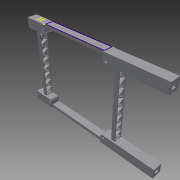
# Autodesk Inventor part: NUCholder
Saved by Autodesk Inventor 2015 (Build 190159000, 159)
## iProperties
Created: 2015-04-17
Part Number: NUCholder
Material: Generic
Document SubType Name: Modeling
Designer: Akovo_000
Density: 1 g/cm^3
Appearance: Default
Author: Akovo_000
Autodesk Inventor part; units mm, degrees
ref_plane "YZ Plane" through (0, 0, 0) normal (1, 0, 0) x (0, 1, 0)
ref_plane "XZ Plane" through (0, 0, 0) normal (0, 1, 0) x (-1, 0, 0)
ref_plane "XY Plane" through (0, 0, 0) normal (0, 0, 1) x (1, 0, 0)
sketch "Button Layer" plane through (0, 0, 0) normal (0, 1, 0) x (-1, 0, 0)
  line L0 (-73.3766, -28.1226) -> (16.7234, -28.1226)
  circle A0 centre (16.7234, -28.1226) radius 1.5
  circle A1 centre (-73.3766, -28.1226) radius 1.5
  line L1 (16.7234, 2.8734) -> (-73.3766, 2.8734)
  circle A2 centre (-11.2766, 30.8734) radius 28
  line L2 (-73.3766, 2.8734) -> (-73.3766, -28.1226)
  line L3 (-73.3766, 47.3774) -> (-73.3766, 2.8734)
  line L4 (16.7234, 2.8734) -> (16.7234, 58.8734)
  line L5 (16.7234, 2.8734) -> (16.7234, -28.1226)
  circle A3 centre (9.7234, -21.1226) radius 3
  circle A4 centre (9.7234, -21.1226) radius 2.5
  line L6 (9.7234, -21.1226) -> (16.7234, -21.1226)
  line L7 (16.7234, -21.1226) -> (16.7234, -28.1226)
  line L8 (16.7234, -28.1226) -> (9.7234, -28.1226)
  line L9 (9.7234, -28.1226) -> (9.7234, -21.1226)
  line L10 (9.7234, -21.1226) -> (-2.2766, -21.1226)
  line L11 (-2.2766, -21.1226) -> (-2.2766, -15.6226)
  line L12 (-2.2766, -15.6226) -> (9.7234, -15.6226)
  line L13 (9.7234, -15.6226) -> (9.7234, -21.1226)
  circle A5 centre (9.7234, -15.6226) radius 2.5
  circle A6 centre (-2.2766, -15.6226) radius 2.5
  line L14 (15.1646, -25.4226) -> (18.2823, -25.4226)
  line L15 (18.2823, -25.4226) -> (19.8411, -28.1226)
  line L16 (19.8411, -28.1226) -> (18.2823, -30.8226)
  line L17 (18.2823, -30.8226) -> (15.1646, -30.8226)
  line L18 (15.1646, -30.8226) -> (13.6057, -28.1226)
  line L19 (13.6057, -28.1226) -> (15.1646, -25.4226)
  line L20 (-74.9354, -25.4226) -> (-71.8177, -25.4226)
  line L21 (-71.8177, -25.4226) -> (-70.2589, -28.1226)
  line L22 (-70.2589, -28.1226) -> (-71.8177, -30.8226)
  line L23 (-71.8177, -30.8226) -> (-74.9354, -30.8226)
  line L24 (-74.9354, -30.8226) -> (-76.4943, -28.1226)
  line L25 (-76.4943, -28.1226) -> (-74.9354, -25.4226)
  line L26 (16.7234, 79.3734) -> (-73.3766, 79.3734)
  line L27 (-73.3766, -15.6266) -> (16.7234, -15.6266)
  circle A7 centre (16.7234, 79.3734) radius 1.5
  circle A8 centre (16.7234, -15.6266) radius 1.5
  circle A9 centre (-73.3766, -15.6266) radius 1.5
  circle A10 centre (-73.3766, 79.3734) radius 1.5
  line L28 (-73.3766, 59.8734) -> (16.7234, 59.8734)
  line L29 (-73.3766, 3.8734) -> (-73.3766, -15.6266)
  line L30 (-73.3766, 59.8734) -> (-73.3766, 79.3734)
  line L31 (-73.3766, 59.8734) -> (-73.3766, 3.8734)
  line L32 (16.7234, 3.8734) -> (16.7234, 59.8734)
  line L33 (16.7234, 3.8734) -> (16.7234, -15.6266)
  circle A11 centre (9.7234, -8.6266) radius 3
  circle A12 centre (9.7234, -8.6266) radius 2.5
  line L34 (9.7234, -8.6266) -> (16.7234, -8.6266)
  line L35 (16.7234, -8.6266) -> (16.7234, -15.6266)
  line L36 (16.7234, -15.6266) -> (9.7234, -15.6266)
  line L37 (9.7234, -15.6266) -> (9.7234, -8.6266)
  line L38 (9.7234, -8.6266) -> (-2.2766, -8.6266)
  line L39 (-2.2766, -8.6266) -> (-2.2766, -3.1266)
  line L40 (-2.2766, -3.1266) -> (9.7234, -3.1266)
  line L41 (9.7234, -3.1266) -> (9.7234, -8.6266)
  circle A13 centre (9.7234, -3.1266) radius 2.5
  circle A14 centre (-2.2766, -3.1266) radius 2.5
  line L42 (15.1646, -12.9266) -> (18.2823, -12.9266)
  line L43 (18.2823, -12.9266) -> (19.8411, -15.6266)
  line L44 (19.8411, -15.6266) -> (18.2823, -18.3266)
  line L45 (18.2823, -18.3266) -> (15.1646, -18.3266)
  line L46 (15.1646, -18.3266) -> (13.6057, -15.6266)
  line L47 (13.6057, -15.6266) -> (15.1646, -12.9266)
  line L48 (15.1646, 82.0734) -> (18.2823, 82.0734)
  line L49 (18.2823, 82.0734) -> (19.8411, 79.3734)
  line L50 (19.8411, 79.3734) -> (18.2823, 76.6734)
  line L51 (18.2823, 76.6734) -> (15.1646, 76.6734)
  line L52 (15.1646, 76.6734) -> (13.6057, 79.3734)
  line L53 (13.6057, 79.3734) -> (15.1646, 82.0734)
  line L54 (-74.9354, 82.0734) -> (-71.8177, 82.0734)
  line L55 (-71.8177, 82.0734) -> (-70.2589, 79.3734)
  line L56 (-70.2589, 79.3734) -> (-71.8177, 76.6734)
  line L57 (-71.8177, 76.6734) -> (-74.9354, 76.6734)
  line L58 (-74.9354, 76.6734) -> (-76.4943, 79.3734)
  line L59 (-76.4943, 79.3734) -> (-74.9354, 82.0734)
  line L60 (-74.9354, -12.9266) -> (-71.8177, -12.9266)
  line L61 (-71.8177, -12.9266) -> (-70.2589, -15.6266)
  line L62 (-70.2589, -15.6266) -> (-71.8177, -18.3266)
  line L63 (-71.8177, -18.3266) -> (-74.9354, -18.3266)
  line L64 (-74.9354, -18.3266) -> (-76.4943, -15.6266)
  line L65 (-76.4943, -15.6266) -> (-74.9354, -12.9266)
  line L66 (41.6234, -38.1226) -> (-138.3766, -38.1226)
  line L67 (-138.3766, -38.1226) -> (-138.3766, 63.8774)
  line L68 (-138.3766, 63.8774) -> (41.6234, 63.8774)
  line L69 (41.6234, 63.8774) -> (41.6234, -38.1226)
  circle A15 centre (-73.3766, -15.6266) radius 3.5
  circle A16 centre (16.7234, -15.6266) radius 3.5
  circle A17 centre (-73.3766, 79.3734) radius 3.5
  circle A18 centre (16.7234, 79.3734) radius 3.5
  line L70 (41.6234, -38.1226) -> (13.2234, -38.1226)
  line L71 (13.2234, -38.1226) -> (13.2234, -12.1266)
  line L72 (13.2234, -12.1266) -> (41.6234, -12.1266)
  line L73 (41.6234, -12.1266) -> (41.6234, -38.1226)
  line L74 (-138.3766, -38.1226) -> (-69.8766, -38.1226)
  line L75 (-69.8766, -38.1226) -> (-69.8766, -12.1266)
  line L76 (-69.8766, -12.1266) -> (-138.3766, -12.1266)
  line L77 (-138.3766, -12.1266) -> (-138.3766, -38.1226)
  line L78 (16.7234, 59.8734) -> (16.7234, 79.3734)
  point P0 (0, 0)
  point P1 (0, 0)
  point P2 (0, 0)
  dimension "d33" = 90.1
  dimension "d35" = 6
  dimension "d36" = 0.5
  dimension "d37" = 5
  dimension "d38" = 12
  dimension "d39" = 7
  dimension "d40" = 5.4
  dimension "d41" = 3
  dimension "d43" = 90.1
  dimension "d45" = 6
  dimension "d46" = 0.5
  dimension "d47" = 5
  dimension "d48" = 12
  dimension "d49" = 7
  dimension "d50" = 5.4
  dimension "d63" = 180
  dimension "d64" = 102
  dimension "d65" = 65
  dimension "d66" = 24.9
  dimension "d67" = 22.496
  dimension "d68" = 7
  dimension "d69" = 10
  dimension "d70" = 57
  constraints: 158 end point, 20 coincident, 19 centre point, 15 parallel, 10 perpendicular, 9 equal length, 9 horizontal, 8 equal radius, 8 tangent, 5 collinear, 4 vertical, 2 concentric, 78 other
  measures "d33" distance of L0.start L0.end
  measures "d35" diameter of A3
  measures "d36" radial gap between concentric circles of A3 A4
  measures "d37" diameter of A5
  measures "d38" distance between parallel lines of L11 L13
  measures "d39" distance of L6.start L6.end
  measures "d40" distance between parallel lines of L15 L18
  measures "d41" diameter of A7
  measures "d43" distance of L27.start L27.end
  measures "d45" diameter of A11
  measures "d46" radial gap between concentric circles of A11 A12
  measures "d47" diameter of A13
  measures "d48" distance between parallel lines of L39 L41
  measures "d49" distance of L34.start L34.end
  measures "d50" distance between parallel lines of L43 L46
  measures "d63" distance of L67.end L68.end
  measures "d64" distance of L66.end L67.end
  measures "d65" distance between parallel lines of L67 L29
  measures "d66" distance between parallel lines of L69 L32
  measures "d67" distance between parallel lines of L66 L27
  measures "d68" diameter of A15
  measures "d69" distance between parallel lines of L66 L0
  measures "d70" distance between parallel lines of L28 L1
sketch "NucSupport" plane through (0, 0, 0) normal (0, 1, 0) x (-1, 0, 0)
  line L0 (0, 0) -> (-180, 0)
  line L1 (-180, 0) -> (-180, 110)
  line L2 (-180, 110) -> (0, 110)
  line L3 (0, 110) -> (0, 0)
  line L4 (-24.9, 8.5) -> (-115, 8.5)
  line L5 (-115, 8.5) -> (-115, 101.5)
  line L6 (-115, 101.5) -> (-24.9, 101.5)
  line L7 (-24.9, 101.5) -> (-24.9, 8.5)
  line L8 (-24.9, 12) -> (0, 12)
  line L9 (-28.4, 8.5) -> (-28.4, 0)
  line L10 (-24.9, 98) -> (0, 98)
  line L11 (-28.4, 101.5) -> (-28.4025, 110)
  line L12 (-111.5, 101.5) -> (-111.5, 110)
  line L13 (-115, 98) -> (-180, 98)
  line L14 (-115, 12) -> (-180, 12)
  line L15 (-111.5, 8.5) -> (-111.5, 0)
  circle A0 centre (-115, 8.5) radius 3.5
  circle A1 centre (-24.9, 8.5) radius 3.5
  circle A2 centre (-115, 101.5) radius 3.5
  circle A3 centre (-24.9, 101.5) radius 3.5
  dimension "d174" = 7
  dimension "d71" = 180
  dimension "d72" = 110
  dimension "d73" = 90.1
  dimension "d74" = 93
  dimension "d75" = 65
  dimension "d176" = 24.9
  constraints: 32 end point, 16 point on line, 9 equal length, 4 coincident, 4 horizontal, 3 vertical, 2 horizontal alignment, 2 vertical alignment, 1 perpendicular, 9 other
  measures "d71" distance of L0.start L0.end
  measures "d72" distance of L0.end L1.end
  measures "d73" distance of L5.end L6.end
  measures "d74" distance of L4.end L5.end
  measures "d75" distance between parallel lines of L1 L5
  measures "d176" distance between parallel lines of L3 L7
extrude "NucSupportHorizontal" add sketch "NucSupport" along normal blind 2 contours L0 L9 A1 L8 L3 | L0 L1 L14 A0 L15 | A1 L7 L4 | L4 L7 A1 | L10 A3 L11 L2 L3 | A0 L5 L4 | L4 L5 A0 | A3 L6 L7 | L7 L6 A3 | L1 L2 L12 A2 L13 | A2 L6 L5 | L5 L6 A2
sketch "Sketch4" plane through (0, 2, 0) normal (0, 1, 0) x (1, 0, 0)
  arc A0 (28.4, -101.5) -> (24.9, -98) centre (24.9, -101.5) ccw projected
  circle A1 centre (24.9, -101.5) radius 3.5
  arc A2 (115, -98) -> (111.5, -101.5) centre (115, -101.5) ccw projected
  circle A3 centre (115, -101.5) radius 3.5
  arc A4 (111.5, -8.5) -> (115, -12) centre (115, -8.5) ccw projected
  circle A5 centre (115, -8.5) radius 3.5
  arc A6 (24.9, -12) -> (28.4, -8.5) centre (24.9, -8.5) ccw projected
  circle A7 centre (24.9, -8.5) radius 3.5
  constraints: 7 equal radius, 4 centre point, 4 coincident
hole "Holes" at (24.9, 2, 101.5) at (24.9, 2, 8.5) at (115, 2, 8.5) at (115, 2, 101.5) direction (0, -1, 0) diameter 3.5 depth 7
sketch "Sketch6" plane through (0, 2, 0) normal (0, 1, 0) x (1, 0, 0)
  line L0 (0, 0) -> (28.4, 0)
  line L1 (28.4, 0) -> (28.4, -8.5)
  line L2 (28.4, -8.5) -> (28.4, 0) projected
  line L3 (24.9, -12) -> (0, -12)
  line L4 (0, -12) -> (0, 0)
  line L5 (0, 0) -> (0, -12) projected
  line L6 (0, -98) -> (24.9, -98)
  line L7 (24.9, -98) -> (0, -98) projected
  line L8 (0, -110) -> (28.4025, -110) projected
  line L9 (28.4025, -110) -> (0, -110)
  line L10 (0, -110) -> (0, -98)
  line L11 (111.5, -110) -> (111.5, -101.5)
  arc A0 (115, -98) -> (111.5, -101.5) centre (115, -101.5) ccw projected
  line L12 (115, -98) -> (180, -98)
  line L13 (180, -98) -> (115, -98) projected
  line L14 (180, -98) -> (180, -110)
  line L15 (180, -110) -> (111.5, -110)
  line L16 (111.5, 0) -> (180, 0)
  line L17 (180, 0) -> (111.5, 0) projected
  line L18 (180, 0) -> (180, -12)
  line L19 (180, -12) -> (115, -12)
  arc A1 (111.5, -8.5) -> (115, -12) centre (115, -8.5) ccw projected
  line L20 (111.5, -8.5) -> (111.5, 0)
  circle A2 centre (115, -101.5) radius 1.75 projected
  arc A3 (115, -98) -> (111.5, -101.5) centre (115, -101.5) ccw
  circle A4 centre (24.9, -8.5) radius 1.75 projected
  arc A5 (24.9, -12) -> (28.4, -8.5) centre (24.9, -8.5) ccw
  circle A6 centre (115, -8.5) radius 1.75 projected
  arc A7 (111.5, -8.5) -> (115, -12) centre (115, -8.5) ccw
  circle A8 centre (24.9, -101.5) radius 1.75 projected
  arc A9 (28.4, -101.5) -> (24.9, -98) centre (24.9, -101.5) ccw
  arc A10 (28.4, -101.5) -> (24.9, -98) centre (24.9, -101.5) ccw projected
  line L21 (28.4, -101.5) -> (28.4025, -110)
  line L22 (0, -12) -> (24.9, -12) projected
  line L23 (28.4025, -110) -> (28.4, -101.5) projected
  line L24 (111.5, -101.5) -> (111.5, -110) projected
  line L25 (111.5, 0) -> (111.5, -8.5) projected
  line L26 (16.9, -12) -> (16.9, -98)
  line L27 (11.9, -98) -> (11.9, -12)
  line L28 (125, -12) -> (125, -98)
  line L29 (180, -98) -> (115, -98) projected
  line L30 (115, -12) -> (180, -12) projected
  line L31 (130, -12) -> (130, -98)
  line L32 (28.4, 0) -> (111.5, 0)
  line L33 (111.5, 0) -> (111.5, -4.25)
  line L34 (111.5, -4.25) -> (28.4, -4.25)
  line L35 (28.4, -4.25) -> (28.4, 0)
  line L36 (111.5, -110) -> (28.4013, -110)
  line L37 (28.4013, -110) -> (28.4013, -105.75)
  line L38 (28.4013, -105.75) -> (111.5, -105.75)
  line L39 (111.5, -105.75) -> (111.5, -110)
  dimension "d179" = 5
  dimension "d181" = 5
  dimension "d183" = 8
  dimension "d184" = 10
  constraints: 56 end point, 9 perpendicular, 9 point on line, 8 point on circle, 7 parallel, 6 collinear, 5 tangent, 4 centre point, 4 coincident, 3 horizontal, 2 midpoint, 1 vertical
  measures "d179" distance between parallel lines of L27 L26
  measures "d181" distance between parallel lines of L31 L28
  measures "d183" distance from line of L26 A5.centre
  measures "d184" distance from line of A7.centre L28
extrude "Big Holder" add sketch "Sketch6" along normal blind 10 contours L0 L1 A5 L3 L4 | L32 L20 L34 L1 | L16 L18 L19 A1 L20 | L3 L26 L6 L27 | L6 A9 L21 L8 L10 | L31 L12 L28 L19 | L12 L14 L15 L11 A0 | L21 L38 L11 L36
sketch "Air Grill" plane through (130, 2, 98) normal (1, 0, 0) x (0, 0, -1)
  line L0 (0, 10) -> (86, 10)
  line L1 (86, 10) -> (86, 0)
  line L2 (86, 0) -> (0, 0)
  line L3 (0, 0) -> (0, 10)
  line L4 (1, 10) -> (85, 10)
  line L5 (85, 10) -> (85, 9.1738)
  line L6 (1, 9.1738) -> (1, 10)
  line L7 (0, 0) -> (86, 0) projected
  line L8 (1, 0) -> (85, 0)
  line L9 (85, 0) -> (85, 1.1182)
  line L10 (1, 0.8262) -> (1, 0)
  line L11 (89.5, 10) -> (86, 10) projected
  line L12 (1, 9.1738) -> (1, 0.8262)
  line L13 (85, 9.1738) -> (85, 1.1182)
  line L14 (86, 0) -> (86, 10) projected
  line L15 (1, 9.1738) -> (5.6509, 1.1182)
  line L16 (1, 9.1738) -> (10.3019, 9.1738) construction
  line L17 (6.4592, 1.1182) -> (11.1102, 9.1738)
  line L18 (6.4592, 1.1182) -> (15.7611, 1.1182) construction
  line L19 (11.9184, 9.1738) -> (16.5694, 1.1182)
  line L20 (17.3777, 1.1182) -> (22.0286, 9.1738)
  line L21 (17.3777, 1.1182) -> (26.6795, 1.1182) construction
  line L22 (22.8369, 9.1738) -> (28.3475, 1.1182)
  line L23 (29.1558, 1.1182) -> (33.8068, 9.1738)
  line L24 (29.1558, 1.1182) -> (38.4577, 1.1182) construction
  line L25 (34.6151, 9.1738) -> (39.266, 1.1182)
  line L26 (34.6151, 9.1738) -> (43.9169, 9.1738) construction
  line L27 (40.0743, 1.1182) -> (44.1917, 9.1738)
  line L28 (11.9184, 9.1738) -> (7.801, 1.1182)
  line L29 (12.7267, 9.1738) -> (17.3777, 1.1182)
  line L30 (18.7195, 1.1182) -> (22.8369, 9.1738)
  line L31 (24.5049, 9.1738) -> (29.1558, 1.1182)
  line L32 (30.4976, 1.1182) -> (34.6151, 9.1738)
  line L33 (35.4234, 9.1738) -> (40.0743, 1.1182)
  line L34 (40.8826, 1.1182) -> (45, 9.1738)
  line L35 (6.4592, 1.1182) -> (5.6509, 1.1182)
  line L36 (16.5694, 1.1182) -> (17.3777, 1.1182)
  line L37 (11.1102, 9.1738) -> (11.9184, 9.1738)
  line L38 (11.9184, 9.1738) -> (11.9184, 9.1738)
  line L39 (12.7267, 9.1738) -> (11.9184, 9.1738)
  line L40 (12.7267, 9.1738) -> (22.0286, 9.1738)
  line L41 (22.0286, 9.1738) -> (22.8369, 9.1738)
  line L42 (22.8369, 9.1738) -> (22.8369, 9.1738)
  line L43 (22.8369, 9.1738) -> (24.5049, 9.1738)
  line L44 (33.8068, 9.1738) -> (24.5049, 9.1738)
  line L45 (33.8068, 9.1738) -> (34.6151, 9.1738)
  line L46 (34.6151, 9.1738) -> (34.6151, 9.1738)
  line L47 (35.4234, 9.1738) -> (34.6151, 9.1738)
  line L48 (35.4234, 9.1738) -> (44.1917, 9.1738)
  line L49 (45, 9.1738) -> (44.1917, 9.1738)
  line L50 (17.3777, 1.1182) -> (17.3777, 1.1182)
  line L51 (16.5694, 1.1182) -> (7.801, 1.1182)
  line L52 (7.801, 1.1182) -> (6.4592, 1.1182)
  line L53 (6.4592, 1.1182) -> (6.4592, 1.1182)
  line L54 (17.3777, 1.1182) -> (18.7195, 1.1182)
  line L55 (18.7195, 1.1182) -> (28.3475, 1.1182)
  line L56 (29.1558, 1.1182) -> (28.3475, 1.1182)
  line L57 (29.1558, 1.1182) -> (29.1558, 1.1182)
  line L58 (29.1558, 1.1182) -> (30.4976, 1.1182)
  line L59 (39.266, 1.1182) -> (30.4976, 1.1182)
  line L60 (39.266, 1.1182) -> (40.0743, 1.1182)
  line L61 (40.0743, 1.1182) -> (40.0743, 1.1182)
  line L62 (40.0743, 1.1182) -> (40.8826, 1.1182)
  line L63 (6.4592, 1.1182) -> (1.8083, 9.1738)
  line L64 (1, 9.1738) -> (1.8083, 9.1738)
  line L65 (11.1102, 9.1738) -> (1.8083, 9.1738)
  line L66 (5.6509, 1.1182) -> (1, 1.1182)
  line L67 (45, 9.1738) -> (49.6509, 1.1182)
  line L68 (45.8083, 9.1738) -> (50.4592, 1.1182)
  line L69 (50.4592, 1.1182) -> (54.5766, 9.1738)
  line L70 (55.3849, 9.1738) -> (60.0359, 1.1182)
  line L71 (56.1932, 9.1738) -> (60.8442, 1.1182)
  line L72 (60.8442, 1.1182) -> (64.9616, 9.1738)
  line L73 (61.6525, 1.1182) -> (65.7699, 9.1738)
  line L74 (65.7699, 9.1738) -> (70.4208, 1.1182)
  line L75 (70.4208, 1.1182) -> (71.2291, 1.1182)
  line L76 (98, -2) -> (98, 10) projected
  line L77 (71.2291, 1.1182) -> (75.3465, 9.1738)
  line L78 (66.5782, 9.1738) -> (71.2291, 1.1182)
  line L79 (71.2291, 1.1182) -> (72.0374, 1.1182)
  line L80 (72.0374, 1.1182) -> (76.1548, 9.1738)
  line L81 (40.8826, 1.1182) -> (49.6509, 1.1182)
  line L82 (0, 10) -> (86, 10) projected
  line L83 (50.4592, 1.1182) -> (49.6509, 1.1182)
  line L84 (50.4592, 1.1182) -> (51.2675, 1.1182)
  line L85 (51.2675, 1.1182) -> (60.0359, 1.1182)
  line L86 (60.0359, 1.1182) -> (60.8442, 1.1182)
  line L87 (60.8442, 1.1182) -> (61.6525, 1.1182)
  line L88 (45, 9.1738) -> (45.8083, 9.1738)
  line L89 (54.5766, 9.1738) -> (45.8083, 9.1738)
  line L90 (55.3849, 9.1738) -> (56.1932, 9.1738)
  line L91 (56.1932, 9.1738) -> (64.9616, 9.1738)
  line L92 (65.7699, 9.1738) -> (64.9616, 9.1738)
  line L93 (65.7699, 9.1738) -> (66.5782, 9.1738)
  line L94 (66.5782, 9.1738) -> (75.3465, 9.1738)
  line L95 (76.1548, 9.1738) -> (75.3465, 9.1738)
  line L96 (55.3849, 9.1738) -> (51.2675, 1.1182)
  line L97 (54.5766, 9.1738) -> (55.3849, 9.1738)
  line L98 (61.6525, 1.1182) -> (70.4208, 1.1182)
  line L99 (76.1548, 9.1738) -> (80.8057, 1.1182)
  line L100 (80.8057, 1.1182) -> (81.614, 1.1182)
  line L101 (86, 10) -> (0, 10) projected
  line L102 (81.614, 1.1182) -> (76.9631, 9.1738)
  line L103 (76.9631, 9.1738) -> (76.1548, 9.1738)
  line L104 (80.8057, 1.1182) -> (72.0374, 1.1182)
  line L105 (81.614, 1.1182) -> (84.1917, 9.1738)
  line L106 (84.1917, 9.1738) -> (76.9631, 9.1738)
  line L107 (0, 0) -> (86, 0) projected
  line L108 (84.1917, 9.1738) -> (85, 9.1738)
  line L109 (86, 0) -> (86, 10) projected
  line L110 (85, 9.1738) -> (82.4223, 1.1182)
  line L111 (81.614, 1.1182) -> (82.4223, 1.1182)
  line L112 (82.4223, 1.1182) -> (85, 1.1182)
  dimension "d185" = 1
  dimension "d186" = 1
  dimension "d188" = 60
  dimension "d189" = 60
  dimension "d191" = 60
  dimension "d193" = 60
  dimension "d194" = 60
  dimension "d197" = 40
  dimension "d198" = 0.7
  dimension "d201" = 0
  dimension "d203" = 1.1182
  constraints: 210 end point, 41 equal length, 33 collinear, 22 parallel, 20 horizontal, 8 point on line, 6 perpendicular, 1 vertical
  measures "d185" distance between parallel lines of L3 L6
  measures "d186" distance between parallel lines of L1 L5
  measures "d188" angle of L15 L16
  measures "d189" angle of L18 L17
  measures "d191" angle of L21 L20
  measures "d193" angle of L24 L23
  measures "d194" angle of L25 L26
  measures "d197" distance of L5.end L34.end
  measures "d198" distance between parallel lines of L63 L15
  measures "d201" distance of L20.start L29.end
  measures "d203" distance between parallel lines of L2 L59
extrude "Extrusion8" cut sketch "Air Grill" against normal blind 120 contours L15 L66 L12 | L13 L112 L110 | L65 L17 L63 | L105 L102 L106 | L28 L19 L51 | L104 L80 L99 | L40 L20 L29 | L77 L78 L94 | L30 L22 L55 | L98 L73 L74 | L44 L23 L31 | L72 L71 L91 | L32 L25 L59 | L85 L96 L70 | L48 L27 L33 | L69 L68 L89 | L34 L67 L81
sketch "Another HOle" plane through (111.5, 0, 110) normal (0, 0, 1) x (1, 0, 0)
  line L0 (-83.0975, 2) -> (0, 2)
  line L1 (0, 2) -> (0, 12)
  line L2 (0, 12) -> (-83.0975, 12)
  line L3 (-83.0975, 12) -> (-83.0975, 2)
  line L4 (-83.1, 12) -> (-83.1, 0) projected
  line L5 (-83.1, 2) -> (-83.1, 12) projected
  line L6 (-94.6, 3.1182) -> (-94.6, 11.1738) projected
  line L7 (-99.6, 3.1182) -> (-99.6, 11.1738) projected
  constraints: 8 end point, 2 parallel, 1 horizontal, 1 perpendicular
sketch "Boss" plane through (0, 12, 0) normal (0, 1, 0) x (1, 0, 0)
  circle A0 centre (24.9, -101.5) radius 1.75 projected
  line L0 (23.3412, -98.8) -> (26.4588, -98.8)
  line L1 (26.4588, -98.8) -> (28.0177, -101.5)
  line L2 (28.0177, -101.5) -> (26.4588, -104.2)
  line L3 (26.4588, -104.2) -> (23.3412, -104.2)
  line L4 (23.3412, -104.2) -> (21.7823, -101.5)
  line L5 (21.7823, -101.5) -> (23.3412, -98.8)
  circle A1 centre (115, -101.5) radius 1.75 projected
  line L6 (116.5588, -98.8) -> (118.1177, -101.5)
  line L7 (118.1177, -101.5) -> (116.5588, -104.2)
  line L8 (116.5588, -104.2) -> (113.4412, -104.2)
  line L9 (113.4412, -104.2) -> (111.8823, -101.5)
  line L10 (111.8823, -101.5) -> (113.4412, -98.8)
  line L11 (113.4412, -98.8) -> (116.5588, -98.8)
  circle A2 centre (115, -8.5) radius 1.75 projected
  line L12 (116.5588, -5.8) -> (118.1177, -8.5)
  line L13 (118.1177, -8.5) -> (116.5588, -11.2)
  line L14 (116.5588, -11.2) -> (113.4412, -11.2)
  line L15 (113.4412, -11.2) -> (111.8823, -8.5)
  line L16 (111.8823, -8.5) -> (113.4412, -5.8)
  line L17 (113.4412, -5.8) -> (116.5588, -5.8)
  circle A3 centre (24.9, -8.5) radius 1.75 projected
  line L18 (26.4588, -5.8) -> (28.0177, -8.5)
  line L19 (28.0177, -8.5) -> (26.4588, -11.2)
  line L20 (26.4588, -11.2) -> (23.3412, -11.2)
  line L21 (23.3412, -11.2) -> (21.7823, -8.5)
  line L22 (21.7823, -8.5) -> (23.3412, -5.8)
  line L23 (23.3412, -5.8) -> (26.4588, -5.8)
  point P0 (0, 0)
  dimension "d232" = 5.4
  constraints: 48 end point, 4 coincident, 3 equal length, 3 parallel, 52 other
  measures "d232" distance between parallel lines of L1 L4
extrude "Extrusion10" cut sketch "Boss" against normal blind 2.4 contours A0 | L0 L1 L2 L3 L4 L5 | L6 L7 L8 L9 L10 L11 | L12 L13 L14 L15 L16 L17 | A3 | L18 L19 L20 L21 L22 L23
sketch "Sketch10" plane through (0, 0, 0) normal (-1, 0, 0) x (0, 0, 1)
  line L0 (98, 12) -> (110, 12)
  line L1 (110, 12) -> (110, 0)
  line L2 (110, 0) -> (98, 0)
  line L3 (98, 0) -> (98, 12)
  line L4 (98, 0) -> (100.5, 0)
  line L5 (100.5, 0) -> (100.5, 2.5)
  line L6 (100.5, 2.5) -> (98, 2.5)
  line L7 (98, 2.5) -> (98, 0)
  line L8 (100.5, 2.5) -> (107.5, 2.5)
  line L9 (107.5, 2.5) -> (107.5, 9.5)
  line L10 (107.5, 9.5) -> (100.5, 9.5)
  line L11 (100.5, 9.5) -> (100.5, 2.5)
  line L12 (107.5, 9.5) -> (110, 9.5)
  line L13 (110, 9.5) -> (110, 12)
  line L14 (110, 12) -> (107.5, 12)
  line L15 (107.5, 12) -> (107.5, 9.5)
  line L16 (0, 12) -> (12, 12)
  line L17 (12, 12) -> (12, 0)
  line L18 (12, 0) -> (0, 0)
  line L19 (0, 0) -> (0, 12)
  line L20 (0, 0) -> (2.5, 0)
  line L21 (2.5, 0) -> (2.5, 2.5)
  line L22 (2.5, 2.5) -> (0, 2.5)
  line L23 (0, 2.5) -> (0, 0)
  line L24 (2.5, 2.5) -> (9.5, 2.5)
  line L25 (9.5, 2.5) -> (9.5, 9.5)
  line L26 (9.5, 9.5) -> (2.5, 9.5)
  line L27 (2.5, 9.5) -> (2.5, 2.5)
  line L28 (12, 12) -> (9.5, 12)
  line L29 (9.5, 12) -> (9.5, 9.5)
  line L30 (9.5, 9.5) -> (12, 9.5)
  line L31 (12, 9.5) -> (12, 12)
  dimension "d238" = 7
  dimension "d239" = 7
  dimension "d240" = 7
  dimension "d241" = 7
  constraints: 64 end point, 16 parallel, 8 horizontal, 8 perpendicular, 6 equal length
  measures "d238" distance between parallel lines of L24 L26
  measures "d239" distance between parallel lines of L27 L25
  measures "d240" distance between parallel lines of L10 L8
  measures "d241" distance between parallel lines of L9 L11
extrude "Extrusion11" cut sketch "Sketch10" against normal blind 5 contours L9 L8 L11 L10 | L25 L24 L27 L26
sketch "Sketch11" plane through (180, 0, 110) normal (1, 0, 0) x (0, 0, -1)
  line L0 (0, 12) -> (12, 12)
  line L1 (12, 12) -> (12, 0)
  line L2 (12, 0) -> (0, 0)
  line L3 (0, 0) -> (0, 12)
  line L4 (110, 0) -> (98, 0)
  line L5 (98, 0) -> (98, 12)
  line L6 (98, 12) -> (110, 12)
  line L7 (110, 12) -> (110, 0)
  line L8 (0, 0) -> (3, 0)
  line L9 (3, 0) -> (3, 3)
  line L10 (3, 3) -> (0, 3)
  line L11 (0, 3) -> (0, 0)
  line L12 (3, 3) -> (9, 3)
  line L13 (9, 3) -> (9, 9)
  line L14 (9, 9) -> (3, 9)
  line L15 (3, 9) -> (3, 3)
  line L16 (12, 12) -> (9, 12)
  line L17 (9, 12) -> (9, 9)
  line L18 (9, 9) -> (12, 9)
  line L19 (12, 9) -> (12, 12)
  line L20 (98, 0) -> (101, 0)
  line L21 (101, 0) -> (101, 3)
  line L22 (101, 3) -> (98, 3)
  line L23 (98, 3) -> (98, 0)
  line L24 (101, 3) -> (107, 3)
  line L25 (107, 3) -> (107, 9)
  line L26 (107, 9) -> (101, 9)
  line L27 (101, 9) -> (101, 3)
  line L28 (110, 12) -> (107, 12)
  line L29 (107, 12) -> (107, 9)
  line L30 (107, 9) -> (110, 9)
  line L31 (110, 9) -> (110, 12)
  dimension "d244" = 6
  dimension "d245" = 6
  dimension "d248" = 12
  dimension "d249" = 12
  constraints: 64 end point, 16 parallel, 8 horizontal, 8 perpendicular, 6 equal length
  measures "d244" distance between parallel lines of L12 L14
  measures "d245" distance between parallel lines of L15 L13
  measures "d248" distance between parallel lines of L3 L1
  measures "d249" distance between parallel lines of L2 L0
extrude "Extrusion12" cut sketch "Sketch11" against normal blind 5 contours L13 L12 L15 L14 | L27 L26 L25 L24
body "Solid3"
